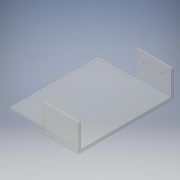
# Autodesk Inventor part: Bucket Top
Saved by Autodesk Inventor 2016 (Build 200138000, 138)
## iProperties
Created: 2015-12-16
Part Number: Bucket Top
Material: PET Plastic
Document SubType Name: Modeling
Designer: TimB
Density: 1.541 g/cm^3
Appearance: Polycarbonate - Clear
Author: TimB
Autodesk Inventor part; units mm, degrees
ref_plane "YZ Plane" through (0, 0, 0) normal (1, 0, 0) x (0, 1, 0)
ref_plane "XZ Plane" through (0, 0, 0) normal (0, 1, 0) x (-1, 0, 0)
ref_plane "XY Plane" through (0, 0, 0) normal (0, 0, 1) x (1, 0, 0)
sketch "Sketch1" plane through (0, 0, 0) normal (0, 1, 0) x (-1, 0, 0)
  line L0 (-50.8, -67.31) -> (50.8, -67.31)
  line L1 (50.8, -67.31) -> (50.8, 67.31)
  line L2 (50.8, 67.31) -> (-50.8, 67.31)
  line L3 (-50.8, 67.31) -> (-50.8, -67.31)
  line L4 (-50.8, -67.31) -> (50.8, 67.31) construction
  line L5 (50.8, -67.31) -> (-50.8, 67.31) construction
  point P0 (0, 0)
  dimension "d0" = 101.6
  dimension "d1" = 134.62
  constraints: 12 end point, 2 midpoint, 2 parallel, 1 horizontal, 1 perpendicular
  measures "d0" distance of L2.end L1.end
  measures "d1" distance of L1.end L0.end
extrude "Extrusion1" add sketch "Sketch1" along normal blind 38.1
sketch "Sketch3" plane through (0, 38.1, 0) normal (0, 1, 0) x (1, 0, 0)
  line L0 (50.8, 63.5) -> (-50.8, 63.5)
  line L1 (-50.8, 63.5) -> (-50.8, -63.5)
  line L2 (-50.8, -63.5) -> (50.8, -63.5)
  line L3 (50.8, -63.5) -> (50.8, 63.5)
  line L4 (50.8, 63.5) -> (-50.8, -63.5) construction
  line L5 (-50.8, 63.5) -> (50.8, -63.5) construction
  point P0 (0, 0)
  dimension "d4" = 127
  constraints: 12 end point, 2 midpoint, 2 parallel, 1 perpendicular
  measures "d4" distance of L1.end L0.end
extrude "Extrusion2" cut sketch "Sketch3" against normal blind 34.29
sketch "Sketch4" plane through (50.8, 0, -67.31) normal (0, 0, -1) x (-1, 0, 0)
  line L0 (101.6, 38.1) -> (50.8, 38.1)
  line L1 (50.8, 38.1) -> (50.8, 0)
  line L2 (50.8, 0) -> (101.6, 0)
  line L3 (101.6, 0) -> (101.6, 38.1)
  dimension "d7" = 50.8
  constraints: 8 end point, 2 parallel, 1 horizontal, 1 perpendicular
  measures "d7" distance of L2.end L1.end
extrude "Extrusion3" cut sketch "Sketch4" against normal blind 5.08
sketch "Sketch5" plane through (-50.8, 0, 67.31) normal (0, 0, 1) x (1, 0, 0)
  line L0 (0, 38.1) -> (0, 3.81) projected
  line L1 (0, 38.1) -> (50.8, 38.1)
  line L2 (50.8, 38.1) -> (50.8, 0)
  line L3 (50.8, 0) -> (0, 0)
  line L4 (0, 0) -> (0, 38.1)
  constraints: 8 end point, 2 parallel, 1 horizontal, 1 perpendicular
extrude "Extrusion4" cut sketch "Sketch5" against normal blind 5.08
sketch "Sketch6" plane through (50.8, 0, 67.31) normal (0, 0, 1) x (1, 0, 0)
  line L0 (-50.8, 38.1) -> (-38.1, 38.1)
  line L1 (-38.1, 38.1) -> (-38.1, 25.4)
  line L2 (-38.1, 25.4) -> (-50.8, 25.4)
  line L3 (-50.8, 25.4) -> (-50.8, 38.1)
  line L4 (0, 38.1) -> (-50.8, 38.1) projected
  line L5 (0, 38.1) -> (-12.7, 38.1)
  line L6 (-12.7, 38.1) -> (-12.7, 25.4)
  line L7 (-12.7, 25.4) -> (0, 25.4)
  line L8 (0, 25.4) -> (0, 38.1)
  point P0 (-50.8, 0)
  dimension "d12" = 12.7
  dimension "d13" = 12.7
  dimension "d14" = 12.7
  constraints: 16 end point, 4 parallel, 2 horizontal, 2 perpendicular
  measures "d12" distance of L1.end L2.end
  measures "d13" distance of L0.end L1.end
  measures "d14" distance of L7.end L6.end
hole "Hole1" at (12.7, 25.4, 67.31) at (38.1, 25.4, 67.31) direction (0, 0, -1) diameter 3.7 end through all
body "Solid1"
